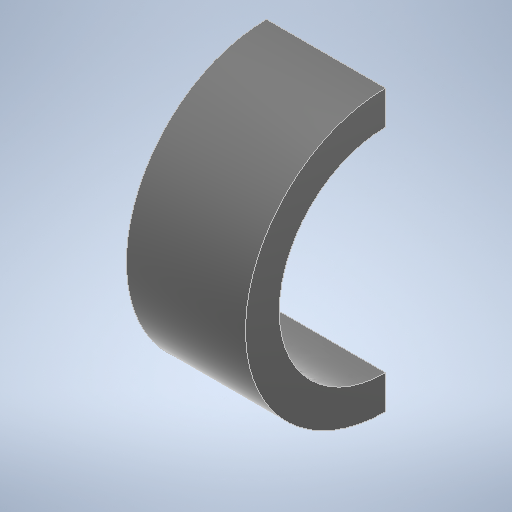
# Autodesk Inventor part: Idler_Pulley_Insert
Saved by Autodesk Inventor 2025.1 (Build 291241020, 241B)
## iProperties
Created: 2024-11-25
Part Number: Idler_Pulley_Insert
Material: ABS Plastic
Document SubType Name: Modeling
Designer: leon-
Density: 1.06 g/cm^3
Appearance: Smooth - Black
Author: leon-
## iProperties of the stored document Idler_Pulley_Insert_3DPrint.ipt
Created: 2024-11-25
Part Number: Idler_Pulley_Insert_3DPrint
Material: Generic
Document SubType Name: Modeling
Designer: leon-
Density: 1 g/cm^3
Appearance: Default
Author: leon-
Autodesk Inventor part; units mm, degrees
ref_plane "YZ Plane" through (0, 0, 0) normal (1, 0, 0) x (0, 1, 0)
ref_plane "XZ Plane" through (0, 0, 0) normal (0, 1, 0) x (-1, 0, 0)
ref_plane "XY Plane" through (0, 0, 0) normal (0, 0, 1) x (1, 0, 0)
sketch "Sketch1" plane through (0, 0, 0) normal (0, 0, 1) x (1, 0, 0)
  line L0 (0, 8) -> (6.8, 8)
  line L1 (6.8, 8) -> (6.8, 6.07)
  line L2 (6.8, 6.07) -> (0, 6.07)
  line L3 (0, 6.07) -> (0, 8)
  line L4 (-1.36, 0) -> (8.16, 0) projected
  point P0 (0, 0)
  point P1 (6.8, 7.035)
  point P2 (0, 7.035)
  dimension "d0" = 6.07
  dimension "d1" = 8
  dimension "d2" = 6.8
  constraints: 8 end point, 2 midpoint, 2 parallel, 1 horizontal, 1 perpendicular, 1 point on line
  measures "d0" distance from line of point (0, 0) L2
  measures "d1" distance from line of point (0, 0) L0
  measures "d2" distance of point (6.8, 7.035) point (0, 7.035)
revolve "Revolution1" add sketch "Sketch1" angle 360 about axis through (-10, 0, 0) along (1, 0, 0)
sketch "Sketch3" plane through (0, 0, 0) normal (0, 0, 1) x (1, 0, 0)
  line L0 (0, -8) -> (0, 8) projected
  line L1 (6.8, -8) -> (6.8, 8) projected
  line L2 (6.8, -6.07) -> (6.8, 6.07) projected
  point P0 (0, 0)
extrude "Extrusion1" cut sketch "Sketch3" against normal through all fills toward (6.75, 0) open curves L2
body "Solid1"
